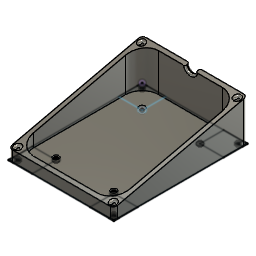
10 Key Main Body v1.1 (Autodesk Fusion 360 design; units mm, degrees)
Autodesk Fusion 360 part; units mm, degrees
sketch "Sketch1" plane through (0, 0, 0) normal (0, 1, 0) x (1, 0, 0)
  line L0 (0, 0) -> (89, 0)
  line L1 (89, 0) -> (89, -113)
  line L2 (89, -113) -> (0, -113)
  line L3 (0, -113) -> (0, 0)
  line L4 (0, 0) -> (4, 0)
  line L5 (4, 0) -> (4, -4)
  line L6 (4, -4) -> (0, -4)
  line L7 (0, -4) -> (0, 0)
  line L8 (89, 0) -> (85, 0)
  line L9 (85, 0) -> (85, -4)
  line L10 (85, -4) -> (89, -4)
  line L11 (89, -4) -> (89, 0)
  line L12 (89, -113) -> (85, -113)
  line L13 (85, -113) -> (85, -109)
  line L14 (85, -109) -> (89, -109)
  line L15 (89, -109) -> (89, -113)
  line L16 (0, -113) -> (4, -113)
  line L17 (4, -113) -> (4, -109)
  line L18 (4, -109) -> (0, -109)
  line L19 (0, -109) -> (0, -113)
  circle A0 centre (4, -4) radius 1.1
  circle A1 centre (85, -4) radius 1.1
  circle A2 centre (85, -109) radius 1.1
  circle A3 centre (4, -109) radius 1.1
  circle A4 centre (20, -20) radius 2.5
  line L20 (89, 0) -> (69, 0)
  line L21 (69, 0) -> (69, -20)
  line L22 (69, -20) -> (89, -20)
  line L23 (89, -20) -> (89, 0)
  line L24 (0, 0) -> (20, 0)
  line L25 (20, 0) -> (20, -20)
  line L26 (20, -20) -> (0, -20)
  line L27 (0, -20) -> (0, 0)
  line L28 (0, -113) -> (20, -113)
  line L29 (20, -113) -> (20, -93)
  line L30 (20, -93) -> (0, -93)
  line L31 (0, -93) -> (0, -113)
  line L32 (89, -113) -> (69, -113)
  line L33 (69, -113) -> (69, -93)
  line L34 (69, -93) -> (89, -93)
  line L35 (89, -93) -> (89, -113)
  circle A5 centre (69, -20) radius 2.5
  circle A6 centre (20, -93) radius 2.5
  circle A7 centre (69, -93) radius 2.5
  dimension "d1" = 89
  dimension "d2" = 113
  dimension "d3" = 4
  dimension "d4" = 4
  dimension "d5" = 4
  dimension "d6" = 4
  dimension "d7" = 4
  dimension "d8" = 4
  dimension "d9" = 4
  dimension "d10" = 4
  dimension "d11" = 2.2
  dimension "d12" = 2.2
  dimension "d13" = 2.2
  dimension "d14" = 2.2
  dimension "d30" = 5
  dimension "d31" = 20
  dimension "d32" = 20
  dimension "d33" = 20
  dimension "d34" = 20
  dimension "d35" = 20
  dimension "d36" = 20
  dimension "d37" = 5
  dimension "d38" = 5
  dimension "d39" = 5
  constraint horizontal L0
  constraint vertical L1
  constraint horizontal L2
  constraint vertical L3
  constraint coincident L0.start L3.end
  constraint horizontal L4
  constraint vertical L5
  constraint horizontal L6
  constraint vertical L7
  constraint horizontal L8
  constraint vertical L9
  constraint horizontal L10
  constraint vertical L11
  constraint horizontal L12
  constraint vertical L13
  constraint horizontal L14
  constraint vertical L15
  constraint horizontal L16
  constraint vertical L17
  constraint horizontal L18
  constraint vertical L19
  constraint coincident L5.end L6.start
  constraint coincident L9.end L10.start
  constraint coincident L13.end L14.start
  constraint coincident L17.end L18.start
  constraint horizontal L20
  constraint vertical L21
  constraint horizontal L22
  constraint vertical L23
  constraint horizontal L24
  constraint vertical L25
  constraint horizontal L26
  constraint vertical L27
  constraint coincident A4.centre L25.end
  constraint horizontal L28
  constraint vertical L29
  constraint horizontal L30
  constraint vertical L31
  constraint horizontal L32
  constraint vertical L33
  constraint horizontal L34
  constraint vertical L35
  constraint coincident L21.end L22.start
  constraint coincident L29.end L30.start
  constraint coincident L33.end L34.start
  measures "d1" distance of L0.start L0.end
  measures "d2" distance of L0.start L2.end
  measures "d3" distance of L0.start L4.end
  measures "d4" distance of L0.start L6.end
  measures "d5" distance of L0.end L8.end
  measures "d6" distance of L0.end L10.end
  measures "d7" distance of L1.end L12.end
  measures "d8" distance of L1.end L14.end
  measures "d9" distance of L2.end L16.end
  measures "d10" distance of L2.end L18.end
  measures "d11" diameter of A0
  measures "d12" diameter of A1
  measures "d13" diameter of A2
  measures "d14" diameter of A3
  measures "d30" diameter of A4
  measures "d31" distance of L0.end L20.end
  measures "d32" distance of L0.end L22.end
  measures "d33" distance of L2.end L28.end
  measures "d34" distance of L2.end L30.end
  measures "d35" distance of L1.end L32.end
  measures "d36" distance of L1.end L34.end
  measures "d37" diameter of A5
  measures "d38" diameter of A6
  measures "d39" diameter of A7
extrude "Extrude1" add sketch "Sketch1" along normal blind 2
sketch "Sketch2" plane through (0, 2, 0) normal (0, 1, 0) x (-1, 0, 0)
  line L0 (0, 0) -> (0, 113)
  line L1 (0, 113) -> (-89, 113)
  line L2 (-89, 113) -> (-89, 0)
  line L3 (-89, 0) -> (0, 0)
  line L4 (0, 0) -> (-89, 0)
  line L5 (-89, 0) -> (-89, 3.5)
  line L6 (-89, 3.5) -> (0, 3.5)
  line L7 (0, 3.5) -> (0, 0)
  line L8 (0, 0) -> (-3.5, 0)
  line L9 (-3.5, 0) -> (-3.5, 113)
  line L10 (-3.5, 113) -> (0, 113)
  line L11 (0, 113) -> (0, 0)
  line L12 (0, 113) -> (-89, 113)
  line L13 (-89, 113) -> (-89, 109.5)
  line L14 (-89, 109.5) -> (0, 109.5)
  line L15 (0, 109.5) -> (0, 113)
  line L16 (-89, 113) -> (-85.5, 113)
  line L17 (-85.5, 113) -> (-85.5, 0)
  line L18 (-85.5, 0) -> (-89, 0)
  line L19 (-89, 0) -> (-89, 113)
  dimension "d17" = 3.5
  dimension "d18" = 3.5
  dimension "d19" = 3.5
  dimension "d20" = 3.5
  constraint horizontal L4
  constraint vertical L5
  constraint horizontal L6
  constraint vertical L7
  constraint coincident L0.start L3.end
  constraint horizontal L8
  constraint vertical L9
  constraint horizontal L10
  constraint vertical L11
  constraint horizontal L12
  constraint vertical L13
  constraint horizontal L14
  constraint vertical L15
  constraint horizontal L16
  constraint vertical L17
  constraint horizontal L18
  constraint vertical L19
  measures "d17" distance of L0.start L6.end
  measures "d18" distance of L0.start L8.end
  measures "d19" distance of L0.end L14.end
  measures "d20" distance of L1.end L16.end
extrude "Extrude2" add sketch "Sketch2" along normal blind 33 contours L0 L3 L4 L6 L7 L8 L9 L11 | L0 L6 L9 L11 L14 | L3 L4 L6 L9 L17 | L0 L1 L9 L10 L11 L12 L14 L15 | L2 L3 L4 L5 L6 L17 L18 L19 | L1 L9 L12 L14 L17 | L2 L6 L14 L17 L19 | L1 L2 L12 L13 L14 L16 L17 L19
sketch "Sketch3" plane through (0, 0, 0) normal (-1, 0, 0) x (0, 0, 1)
  line L0 (0, 0) -> (113, 0)
  line L1 (113, 0) -> (113, 35)
  line L2 (113, 35) -> (0, 35)
  line L3 (0, 35) -> (0, 0)
  line L4 (113, 0) -> (113, 9)
  line L5 (113, 9) -> (0, 35)
  dimension "d23" = 9
  constraint coincident L0.end L1.start
  constraint perpendicular L0 L4
  constraint coincident L2.end L3.start
  measures "d23" distance of L0.end L4.end
extrude "Extrude3" cut sketch "Sketch3" against normal blind 92 contours L1 L2 L5
fillet "Fillet1" radius 14 4 edges at (3.5, 18.0973, 3.5) (85.5, 18.0973, 3.5) (85.5, 5.9027, 109.5) (3.5, 5.9027, 109.5)
extrude "Extrude4" cut sketch "Sketch1" along normal blind 50 contours L5 L6 A0 | L5 L6 A0 | L9 L10 A1 | L9 L10 A1 | L17 L18 A3 | L17 L18 A3 | L13 L14 A2 | L13 L14 A2
extrude "Extrude5" cut sketch "Sketch1" along normal blind 5 contours A4 L25 L26 | A4 L25 L26 | L21 L22 A5 | L21 L22 A5 | L29 L30 A6 | L29 L30 A6 | L33 L34 A7 | L33 L34 A7
fillet "Fillet2" radius 3 4 edges at (0, 4.5, 113) (89, 4.5, 113) (89, 17.5, 0) (0, 17.5, 0)
fillet "Fillet3" radius 2 4 edges at (4, 9.6673, 110.1) (85, 9.6673, 110.1) (85, 33.8265, 5.1) (4, 33.8265, 5.1)
sketch "Sketch4" plane through (0, 0, 0) normal (0, 0, -1) x (-1, 0, 0)
  line L0 (-3, 0) -> (-3, 35)
  line L1 (-3, 35) -> (-86, 35)
  line L2 (-86, 35) -> (-86, 0)
  line L3 (-86, 0) -> (-3, 0)
  line L4 (-86, 35) -> (-44.5, 35)
  circle A0 centre (-44.5, 35) radius 4.5
  constraint coincident L1.end L2.start
  constraint midpoint L1 L4.end
  constraint coincident L4.end A0.centre
extrude "Extrude6" cut sketch "Sketch4" against normal blind 6 contours L1 L4 A0 picked at (-47.4832, 34.7764)
fillet "Fillet4" radius 1.5 2 edges at (44.5, 30.5, 0) (44.5, 30.5, 3.5)
